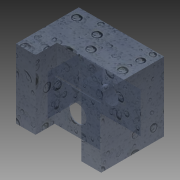
# Autodesk Inventor part: MudGuardBrace
Saved by Autodesk Inventor 2014 SP1 (Build 180222100, 222)
## iProperties
Created: 2017-01-24
Part Number: MudGuardBrace
Material: Generic
Document SubType Name: Modeling
Designer: danielsikar
Density: 1 g/cm^3
Appearance: Water Bubbles
Author: danielsikar
Autodesk Inventor part; units mm, degrees
ref_plane "YZ Plane" through (0, 0, 0) normal (1, 0, 0) x (0, 1, 0)
ref_plane "XZ Plane" through (0, 0, 0) normal (0, 1, 0) x (-1, 0, 0)
ref_plane "XY Plane" through (0, 0, 0) normal (0, 0, 1) x (1, 0, 0)
sketch "Sketch1" plane through (0, 0, 0) normal (0, 0, 1) x (1, 0, 0)
  line L0 (0, 0) -> (21, 0)
  line L1 (21, 0) -> (21, 15.5)
  line L2 (21, 15.5) -> (0, 15.5)
  line L3 (0, 15.5) -> (0, 0)
  dimension "d0" = 21
  dimension "d1" = 15.5
  constraints: 8 end point, 2 parallel, 1 horizontal, 1 perpendicular
  measures "d0" distance of L2.end L1.end
  measures "d1" distance of L1.end L0.end
extrude "Extrusion1" add sketch "Sketch1" along normal blind 17
sketch "Sketch3" plane through (0, 15.5, 0) normal (0, 1, 0) x (1, 0, 0)
  arc A0 (10.5, -7.15) -> (10.5, -2.85) centre (10.5, -5) ccw projected
  arc A1 (10.5, -2.85) -> (10.5, -7.15) centre (10.5, -5) ccw projected
extrude "Extrusion2" cut sketch "Sketch3" against normal through all
sketch "Sketch5" plane through (0, 0, 0) normal (0, 0, -1) x (-1, 0, 0)
  line L0 (0, 0) -> (-21, 0) projected
  line L1 (-16.3094, 5.2919) -> (-4.6578, 5.2919)
  line L2 (-4.6578, 5.2919) -> (-4.6578, 0)
  line L3 (-4.6578, 0) -> (-16.3094, 0)
  line L4 (-16.3094, 0) -> (-16.3094, 5.2919)
  constraints: 8 end point, 2 parallel, 1 horizontal, 1 perpendicular, 1 point on line
extrude "Extrusion3" cut sketch "Sketch5" against normal through all
ref_plane "Work Plane1" through (0, 0, 10) normal (0, 0, 1) x (1, 0, 0)
sketch "Sketch6" plane through (0, 0, 10) normal (0, 0, 1) x (1, 0, 0)
  line L0 (3, 12.5) -> (10.5, 12.5) projected
  line L1 (18, 12.5) -> (10.5, 12.5) projected
  line L2 (18, 5) -> (18, 12.5) projected
  line L3 (3, 5) -> (3, 12.5) projected
  line L4 (10.5, 5) -> (3, 5) projected
  line L5 (10.5, 5) -> (18, 5) projected
  line L6 (10.5, 12.8) -> (2.7, 12.8)
  line L7 (2.7, 12.8) -> (2.7, 4.7)
  line L8 (2.7, 4.7) -> (10.5, 4.7)
  line L9 (10.5, 4.7) -> (18.3, 4.7)
  line L10 (18.3, 4.7) -> (18.3, 12.8)
  line L11 (18.3, 12.8) -> (10.5, 12.8)
  point P0 (0, 0)
  dimension "d10" = 0.3
  constraints: 12 end point, 5 other
  measures "d10" distance between parallel lines of L10 L2
ref_plane "Work Plane2" through (3, 12.5, 0) normal (0, 0, 1) x (1, 0, 0)
extrude "Extrusion4" add sketch "Sketch6" against normal up to surface (10 mm away) contours L0 L1 L2 L5 L4 L3 | L11 L10 L9 L8 L7 L6
sketch "Sketch7" plane through (10.5, 12.8, 5) normal (0, 1, 0) x (1, 0, 0)
  circle A0 centre (0, 0) radius 2.15 projected
  point P0 (-10.5, 5)
extrude "Extrusion5" cut sketch "Sketch7" against normal blind 10
sketch "Sketch10" plane through (0, 0, 10) normal (0, 0, 1) x (1, 0, 0)
  line L0 (18, 5) -> (18, 12.5)
  line L1 (18, 12.5) -> (10.5, 12.5)
  line L2 (3, 5) -> (3, 12.5)
  line L3 (10.5, 5) -> (3, 5)
  line L4 (10.5, 5) -> (18, 5)
  line L5 (3, 12.5) -> (10.5, 12.5)
  line L6 (10.5, 12.6) -> (18.1, 12.6)
  line L7 (18.1, 12.6) -> (18.1, 4.9)
  line L8 (18.1, 4.9) -> (10.5, 4.9)
  line L9 (10.5, 4.9) -> (2.9, 4.9)
  line L10 (2.9, 4.9) -> (2.9, 12.6)
  line L11 (2.9, 12.6) -> (10.5, 12.6)
  point P0 (0, 0)
  dimension "d15" = 0.1
  constraints: 24 end point, 4 horizontal, 2 vertical, 11 other
  measures "d15" distance between parallel lines of L11 L5
ref_plane "Work Plane3" through (3, 12.5, 0) normal (0, 0, 1) x (1, 0, 0)
extrude "Extrusion6" cut sketch "Sketch10" against normal up to surface (10 mm away) contours L4 L3 L2 L5 L1 L0 | L6 L7 L8 L9 L10 L11
sketch "Sketch11" plane through (4.6578, 0, 17) normal (1, 0, 0) x (0, 0, -1)
  line L0 (7, 4.7) -> (7, 4.9) projected
  line L1 (7, 4.9) -> (7, 5.2919) projected
  line L2 (7, 5.2919) -> (0, 5.2919) projected
  line L3 (0, 0) -> (0, 5.2919) projected
  line L4 (17, 0) -> (0, 0) projected
  line L5 (17, 4.7) -> (17, 0) projected
  line L6 (17, 4.7) -> (7, 4.7) projected
extrude "Extrusion7" add sketch "Sketch11" along normal blind 0.2
sketch "Sketch12" plane through (16.3094, 0, 17) normal (-1, 0, 0) x (0, 0, 1)
  line L0 (-7, 4.7) -> (-17, 4.7) projected
  line L1 (-17, 0) -> (-17, 4.7) projected
  line L2 (0, 0) -> (-17, 0) projected
  line L3 (0, 5.2919) -> (0, 0) projected
  line L4 (-7, 5.2919) -> (0, 5.2919) projected
  line L5 (-7, 5.2919) -> (-7, 4.9) projected
  line L6 (-7, 4.9) -> (-7, 4.7) projected
extrude "Extrusion8" add sketch "Sketch12" along normal blind 0.2
body "Solid1"
